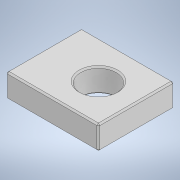
# Autodesk Inventor part: Calza para ventilador
Saved by Autodesk Inventor 2020.5 (Build 245400000, 400)
## iProperties
Created: 2022-04-13
Part Number: Calza para ventilador
Material: Generic
Document SubType Name: Modeling
Designer: aivel
Density: 1 g/cm^3
Appearance: Default
Author: aivel
Autodesk Inventor part; units mm, degrees
ref_plane "YZ Plane" through (0, 0, 0) normal (1, 0, 0) x (0, 1, 0)
ref_plane "XZ Plane" through (0, 0, 0) normal (0, 1, 0) x (-1, 0, 0)
ref_plane "XY Plane" through (0, 0, 0) normal (0, 0, 1) x (1, 0, 0)
sketch "Sketch1" plane through (0, 0, 0) normal (0, 1, 0) x (-1, 0, 0)
  line L0 (0, 0) -> (-15.85, 0) construction
  line L1 (-15.85, 0) -> (-15.85, -13) construction
  line L2 (-15.85, -13) -> (0, -13) construction
  line L3 (0, -13) -> (0, 0) construction
  line L4 (0, 0) -> (-9.35, 0) construction
  line L5 (-9.35, 0) -> (-9.35, -6.5) construction
  line L6 (-9.35, -6.5) -> (0, -6.5) construction
  line L7 (0, -6.5) -> (0, 0) construction
  circle A0 centre (-9.35, -6.5) radius 3
  line L8 (0, 0) -> (-0.15, 0) construction
  line L9 (-0.15, 0) -> (-0.15, -0.15) construction
  line L10 (-0.15, -0.15) -> (0, -0.15) construction
  line L11 (0, -0.15) -> (0, 0) construction
  line L12 (-15.85, -13) -> (-15.7, -13) construction
  line L13 (-15.7, -13) -> (-15.7, -12.85) construction
  line L14 (-15.7, -12.85) -> (-15.85, -12.85) construction
  line L15 (-15.85, -12.85) -> (-15.85, -13) construction
  line L16 (-0.15, -0.15) -> (-15.7, -0.15)
  line L17 (-15.7, -0.15) -> (-15.7, -12.85)
  line L18 (-15.7, -12.85) -> (-0.15, -12.85)
  line L19 (-0.15, -12.85) -> (-0.15, -0.15)
  dimension "d0" = 15.85
  dimension "d1" = 13
  dimension "d2" = 9.35
  dimension "d3" = 6.5
  dimension "d4" = 6
  constraints: 40 end point, 10 parallel, 5 horizontal, 5 perpendicular, 1 centre point, 1 coincident
  measures "d0" distance of L2.end L1.end
  measures "d1" distance of L1.end L0.end
  measures "d2" distance of L6.end L5.end
  measures "d3" distance of L5.end L4.end
  measures "d4" diameter of A0
extrude "Extrusion1" add sketch "Sketch1" along normal blind 4
chamfer "Chamfer1" distance 0.25 angle 45 14 edges at (0.15, 4, -6.5) (7.925, 4, -12.85) (15.7, 4, -6.5) (7.925, 4, -0.15) (0.15, 2, -0.15) (15.7, 2, -0.15) (15.7, 2, -12.85) (0.15, 2, -12.85) (0.15, 0, -6.5) (7.925, 0, -12.85) (12.35, 4, -6.5) (12.35, 0, -6.5) (15.7, 0, -6.5) (7.925, 0, -0.15)
body "Solid1"
